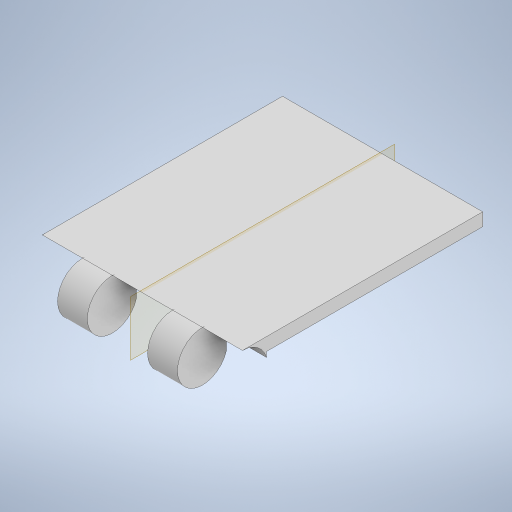
# Autodesk Inventor part: knuckle plate hinge 2
Saved by Autodesk Inventor 2024.2 (Build 282272000, 272)
## iProperties
Created: 2024-11-15
Part Number: knuckle plate hinge 2
Material: Generic
Document SubType Name: Modeling
Designer: Tom
Density: 1 g/cm^3
Appearance: Default
Author: Tom
Autodesk Inventor part; units mm, degrees
ref_plane "XZ Plane" through (0, 0, 0) normal (0, 1, 0) x (-1, 0, 0)
ref_plane "XY Plane" through (0, 0, 0) normal (0, 0, 1) x (1, 0, 0)
sketch "Sketch1" plane through (0, 0, 0) normal (0, 1, 0) x (-1, 0, 0)
  line L0 (0, 0) -> (63.5, 0)
  line L1 (63.5, 0) -> (63.5, -76.2)
  line L2 (63.5, -76.2) -> (0, -76.2)
  line L3 (0, -76.2) -> (0, 0)
  dimension "d0" = 63.5
  dimension "d1" = 76.2
  constraints: 8 end point, 2 parallel, 1 horizontal, 1 perpendicular
  measures "d0" distance of L0.start L0.end
  measures "d1" distance of L2.end L0.start
extrude "Extrusion1" add sketch "Sketch1" along normal blind 15.875
sketch "Sketch2" plane through (0, 0, 0) normal (1, 0, 0) x (0, 0, -1)
  line L0 (76.2, 0) -> (0, 0) projected
  line L1 (0, 0) -> (0, 15.875) projected
  circle A0 centre (0, 7.9375) radius 7.9375
  line L2 (76.2, 15.875) -> (0, 15.875) projected
  constraints: 1 centre point, 1 midpoint, 1 tangent
extrude "Extrusion2" cut sketch "Sketch2" against normal blind 12.7 contours L1 A0 picked at (1.148, 10.3213)
ref_plane "Work Plane1" through (-31.75, 0, 0) normal (1, 0, 0) x (0, 1, 0)
mirror "Mirror1" about plane through (-31.75, 0, 0) normal (1, 0, 0) of "Extrusion2"
sketch "Sketch3" plane through (-12.7, 0, 0) normal (0, 0, 1) x (1, 0, 0)
  line L0 (12.7, 15.875) -> (-50.8, 15.875) projected
  line L1 (12.7, 0) -> (-50.8, 0) projected
  line L2 (-28.575, 15.875) -> (-9.525, 15.875)
  line L3 (-9.525, 15.875) -> (-9.525, 7.9375)
  line L4 (-28.575, 7.9375) -> (-28.575, 15.875)
  line L5 (0, 0) -> (0, 15.875) projected
  line L6 (-28.575, 7.9375) -> (-9.525, 7.9375)
  line L7 (-32.6367, 7.9375) -> (-5.0262, 7.9375)
  point P0 (-9.525, 15.875)
  dimension "d8" = 19.05
  dimension "d9" = 9.525
  constraints: 10 end point, 2 point on line, 1 horizontal, 1 parallel, 1 perpendicular
  measures "d8" distance between parallel lines of L4 L3
  measures "d9" distance between parallel lines of L5 L3
revolve "Revolution1" cut sketch "Sketch3" angle 360 about axis through (-45.3367, 7.9375, 0) along (1, 0, 0)
sketch "Sketch4" plane through (-12.7, 0, 0) normal (0, 0, 1) x (1, 0, 0)
  line L0 (12.7, 15.875) -> (-50.8, 15.875) projected
  line L1 (0, 0) -> (0, 15.875) projected
  line L2 (-9.4737, 15.875) -> (0, 15.875)
  line L3 (0, 15.875) -> (0, 7.9375)
  line L4 (0, 7.9375) -> (-9.4737, 7.9375)
  line L5 (-9.4737, 7.9375) -> (-9.4737, 15.875)
  line L6 (-28.575, 15.875) -> (-28.575, 0) projected
  line L7 (-38.032, 15.875) -> (-28.575, 15.875)
  line L8 (-28.575, 15.875) -> (-28.575, 7.9375)
  line L9 (-28.575, 7.9375) -> (-38.032, 7.9375)
  line L10 (-38.032, 7.9375) -> (-38.032, 15.875)
  line L11 (-38.032, 7.9375) -> (0, 7.9375)
  point P0 (12.7, 0)
  constraints: 18 end point, 4 parallel, 3 horizontal, 2 midpoint, 2 perpendicular, 2 point on line
revolve "Revolution2" add sketch "Sketch4" angle 360 about axis through (-50.732, 7.9375, 0) along (1, 0, 0) contours L1 L4 L5 L0 | L6 L9 L10 L0
sketch "Sketch5" plane through (0, 0, -76.2) normal (1, 0, 0) x (0, 0, -1)
  line L0 (0, 0) -> (0, 15.875) projected
  line L1 (0, 0) -> (-63.4859, 0)
  line L2 (-63.4859, 0) -> (-63.4859, -0.635)
  line L3 (-63.4859, -0.635) -> (0, -0.635)
  line L4 (0, -0.635) -> (0, 0)
  line L5 (-76.2, 15.875) -> (0, 15.875) projected
  point P0 (-76.2, 0)
  dimension "d12" = 16.51
  constraints: 8 end point, 2 parallel, 1 horizontal, 1 perpendicular
  measures "d12" distance between parallel lines of L3 L5
extrude "Extrusion3" add sketch "Sketch5" against normal up to surface (63.5 mm away)
sketch "Sketch6" plane through (0, 7.9375, 0) normal (1, 0, 0) x (0, 0, -1)
  line L0 (12.7141, -8.5725) -> (76.2, -8.5725) projected
  line L1 (76.2, -8.5725) -> (7.62, -8.5725)
  line L2 (7.62, -8.5725) -> (7.62, 3.8481)
  line L3 (7.62, 3.8481) -> (76.2, 3.8481)
  line L4 (76.2, 3.8481) -> (76.2, -8.5725)
  line L5 (0, 7.9375) -> (76.2, 7.9375) projected
  point P0 (0, -7.9375)
  dimension "d15" = 4.0894
  dimension "d16" = 68.58
  constraints: 8 end point, 2 parallel, 1 horizontal, 1 perpendicular
  measures "d15" distance between parallel lines of L3 L5
  measures "d16" distance of L2.end L3.end
extrude "Extrusion4" cut sketch "Sketch6" against normal through all
sketch "Sketch7" plane through (0, 0, 0) normal (1, 0, 0) x (0, 0, -1)
  arc A0 (0, 0) -> (7.62, 5.715) centre (0, 7.9375) ccw projected
  line L0 (7.62, 5.715) -> (7.62, 0)
  line L1 (7.62, 0) -> (0, 0)
  arc A1 (0, 0) -> (7.62, 5.715) centre (0, 7.9375) ccw
  constraints: 4 end point, 2 point on circle, 1 centre point, 1 concentric, 1 perpendicular
extrude "Extrusion5" cut sketch "Sketch7" against normal through all
body "Solid1"
